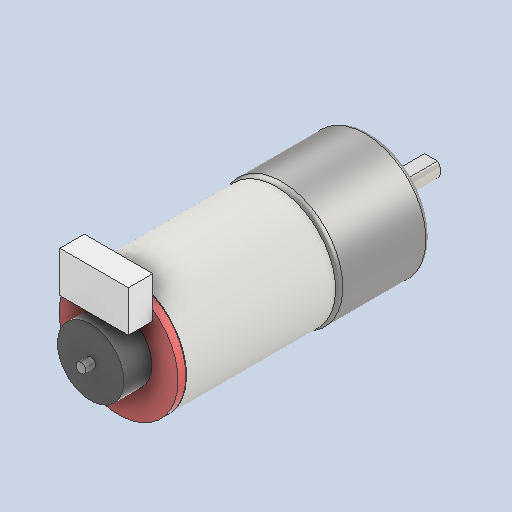
# Autodesk Inventor part: servo
Saved by Autodesk Inventor 2023 (Build 270158000, 158)
## iProperties
Created: 2023-03-11
Part Number: servo
Material: Типовые
Document SubType Name: Modeling
Designer: Khasal
Density: 1 g/cm^3
Appearance: По умолчанию
Author: Khasal
Autodesk Inventor part; units mm, degrees
ref_plane "YZ Plane" through (0, 0, 0) normal (1, 0, 0) x (0, 1, 0)
ref_plane "XZ Plane" through (0, 0, 0) normal (0, 1, 0) x (-1, 0, 0)
ref_plane "XY Plane" through (0, 0, 0) normal (0, 0, 1) x (1, 0, 0)
sketch "Эскиз1" plane through (0, 0, 0) normal (1, 0, 0) x (0, 1, 0)
  line L0 (0, 0) -> (11.15, 0)
  line L1 (12.15, 0.134) -> (12.15, 30.616)
  line L2 (12.15, 30.75) -> (11.65, 30.75)
  line L3 (11.65, 30.75) -> (12.15, 30.616)
  line L4 (11.65, 30.75) -> (12.7154, 30.75) construction
  line L5 (12.15, 30.75) -> (12.15, 32.35)
  line L6 (12.15, 32.35) -> (0, 32.35)
  line L7 (11.65, 30.75) -> (0, 30.75)
  line L8 (0, 32.35) -> (0, 0)
  line L9 (12.15, 0) -> (11.65, 0)
  line L10 (11.65, 0) -> (12.15, 0.134)
  line L11 (0, 32.35) -> (6.8, 32.35)
  line L12 (6.8, 32.35) -> (6.8, 38.05)
  line L13 (6.8, 38.05) -> (0, 38.05)
  line L14 (0, 38.05) -> (0, 32.35)
  line L15 (0, 38.05) -> (0, 40.05)
  line L16 (0, 40.05) -> (1, 40.05)
  line L17 (1, 40.05) -> (1, 38.05)
  line L18 (11.65, 0) -> (12.15, 0)
  line L19 (0, 0) -> (0, -19)
  line L20 (0, -19) -> (0, -21.75)
  line L21 (0, -21.75) -> (3.5, -21.75)
  line L22 (3.5, -21.75) -> (3.5, -19)
  line L23 (0, -21.75) -> (2, -21.75)
  line L24 (2, -21.75) -> (2, -31.55)
  line L25 (2, -31.55) -> (0, -31.55)
  line L26 (0, -31.55) -> (0, -21.75)
  line L27 (11.65, 0) -> (11.15, 0)
  line L28 (0, -19) -> (11.5, -19)
  line L29 (12.5, -18) -> (12.5, -1)
  line L30 (11.5, 0) -> (11.65, 0)
  arc A0 (12.5, -1) -> (11.5, 0) centre (11.5, -1) ccw
  arc A1 (11.5, -19) -> (12.5, -18) centre (11.5, -18) ccw
  point P0 (12.5, -19)
  dimension "d0" = 12.15
  dimension "d1" = 30.75
  dimension "d2" = 0.5
  dimension "d4" = 15
  dimension "d5" = 1.6
  dimension "d6" = 0.5
  dimension "d7" = 15
  dimension "d8" = 6.8
  dimension "d9" = 5.7
  dimension "d10" = 2
  dimension "d11" = 1
  dimension "d13" = 2.75
  dimension "d14" = 3.5
  dimension "d15" = 2
  dimension "d16" = 9.8
  dimension "d23" = 12.5
  dimension "d24" = 1
  constraints: 62 end point, 14 perpendicular, 7 point on line, 4 horizontal, 4 point on circle, 4 tangent, 4 vertical, 3 collinear, 2 centre point, 1 equal radius
  measures "d0" distance of L0.start L9.start
  measures "d1" distance of L9.start L2.start
  measures "d2" distance of L2.start L2.end
  measures "d4" angle of L3 L4
  measures "d5" distance of L2.start L5.end
  measures "d6" distance of L9.start L9.end
  measures "d7" angle of L9 L10
  measures "d8" distance of L6.end L11.end
  measures "d9" distance of L11.end L12.end
  measures "d10" distance of L13.end L15.end
  measures "d11" distance of L15.end L16.end
  measures "d13" distance of L19.end L20.end
  measures "d14" distance of L20.end L21.end
  measures "d15" distance of L20.end L23.end
  measures "d16" distance of L23.end L24.end
  measures "d23" distance of L19.end point (12.5, -19)
  measures "d24" radius of A0
revolve "Вращение1" add sketch "Эскиз1" angle 360 about axis through (0, 0, 38.05) along (0, 0, 1) contours L15 L16 L17 L13
revolve "Вращение2" add sketch "Эскиз1" angle 360 about axis through (0, 0, 38.05) along (0, 0, -1) contours L14 L13 L12 L6
revolve "Вращение3" add sketch "Эскиз1" angle 360 about axis through (0, 0, 32.35) along (0, 0, -1) contours L8 L6 L5 L2 L7
revolve "Вращение4" add sketch "Эскиз1" angle 360 about axis through (0, 0, 32.35) along (0, 0, -1) contours L8 L7 L3 L1 L10 L27 L0
revolve "Вращение5" add sketch "Эскиз1" angle 360 about axis through (0, 0, 0) along (0, 0, -1) contours L0 L27 A0 L29 A1 L28 L19
revolve "Вращение6" add sketch "Эскиз1" angle 360 about axis through (0, 0, -19) along (0, 0, -1) contours L28 L22 L21 L20
revolve "Вращение7" add sketch "Эскиз1" angle 360 about axis through (0, 0, -31.55) along (0, 0, 1) contours L21 L24 L25 L26
sketch "Эскиз2" plane through (0, 0, 32.35) normal (0, 0, 1) x (1, 0, 0)
  line L0 (-7, 7.95) -> (7, 7.95)
  line L1 (7, 7.95) -> (7, 16.35)
  line L2 (7, 16.35) -> (-7, 16.35)
  line L3 (-7, 16.35) -> (-7, 7.95)
  line L4 (-7, 7.95) -> (7, 16.35) construction
  line L5 (7, 7.95) -> (-7, 16.35) construction
  circle A0 centre (0, 0) radius 12.15 projected
  point P0 (0, 12.15)
  dimension "d28" = 14
  dimension "d29" = 8.4
  constraints: 12 end point, 2 midpoint, 2 parallel, 1 horizontal, 1 perpendicular, 1 vertical alignment, 1 other
  measures "d28" distance of L1.end L2.end
  measures "d29" distance of L0.end L1.end
extrude "Выдавливание1" add sketch "Эскиз2" along normal blind 5 contours L3 A0 L1 L0 | L3 L2 L1 A0 picked at (-0.4961, 9.3195)
sketch "Эскиз3" plane through (0, 0, -31.55) normal (0, 0, -1) x (-1, 0, 0)
  line L0 (-1.8903, 1.5) -> (1.8903, 1.5)
  line L1 (1.8903, 1.5) -> (1.8903, 3.1362)
  line L2 (1.8903, 3.1362) -> (-1.8903, 3.1362)
  line L3 (-1.8903, 3.1362) -> (-1.8903, 1.5)
  line L4 (-1.8903, 1.5) -> (1.8903, 3.1362) construction
  line L5 (1.8903, 1.5) -> (-1.8903, 3.1362) construction
  circle A0 centre (0, 0) radius 2 projected
  point P0 (0, 2.3181)
  dimension "d32" = 1.5
  constraints: 12 end point, 2 midpoint, 2 parallel, 1 horizontal, 1 perpendicular
  measures "d32" distance from line of point (0, 0) L0
extrude "Выдавливание2" cut sketch "Эскиз3" against normal blind 8.55 contours L3 L2 L1 L0 A0 | A0 L0 picked at (0, 1.6667)
sketch "Эскиз4" plane through (0, 0, -19) normal (0, 0, -1) x (-1, 0, 0)
  circle A0 centre (0, 0) radius 3.5 projected
  circle A1 centre (0, 0) radius 11.5 projected
  circle A2 centre (0, 8.5) radius 0.4758
  line L0 (-17.5, 0) -> (17.5, 0) projected
  circle A3 centre (0, -8.5) radius 0.4758
  dimension "d35" = 8.5
  constraints: 2 centre point, 1 symmetric about line, 1 other
  measures "d35" distance from line of L0 A2.centre
hole "Отверстие1" at (0, 8.5, -19) at (0, -8.5, -19) direction (0, 0, 1) diameter 2.459 depth 11.5 tip angle 118 countersink diameter 3.5 countersink angle 90 thread size "M3x0.5" class "6H" standard "ISO Metric profile"
